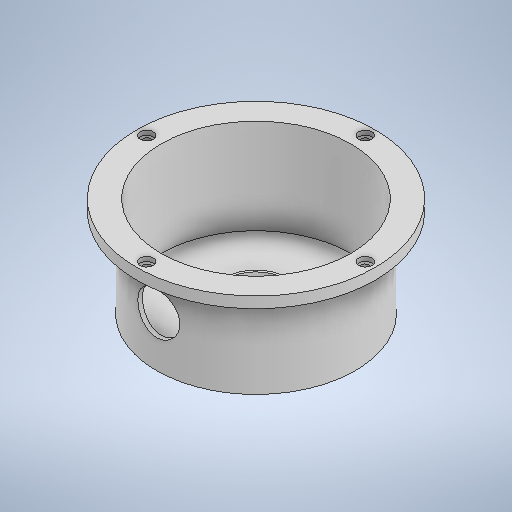
# Autodesk Inventor part: Pieza 3
Saved by Autodesk Inventor 2025.1 (Build 291241000, 241)
## iProperties
Created: 2024-08-11
Part Number: Pieza 3
Material: Genérico
Document SubType Name: Modeling
Designer: andre
Density: 1 g/cm^3
Appearance: Valor por defecto
Author: andre
Autodesk Inventor part; units mm, degrees
ref_plane "YZ Plane" through (0, 0, 0) normal (1, 0, 0) x (0, 1, 0)
ref_plane "XZ Plane" through (0, 0, 0) normal (0, 1, 0) x (-1, 0, 0)
ref_plane "XY Plane" through (0, 0, 0) normal (0, 0, 1) x (1, 0, 0)
sketch "Boceto1" plane through (0, 0, 0) normal (0, 1, 0) x (-1, 0, 0)
  circle A0 centre (0, 0) radius 45
  circle A1 centre (0, 0) radius 54
  circle A2 centre (0, 0) radius 43
  dimension "d0" = 90
  dimension "d1" = 9
  dimension "d8" = 2
  constraints: 3 centre point, 1 coincident
  measures "d0" diameter of A0
  measures "d1" radial gap between concentric circles of A0 A1
  measures "d8" radial gap between concentric circles of A0 A2
extrude "Extrusión1" add sketch "Boceto1" along normal blind 5 contours A0 | A1
sketch "Boceto2" plane through (0, 0, 0) normal (0, -1, 0) x (1, 0, 0)
  circle A0 centre (0, 0) radius 45
  circle A1 centre (0, 0) radius 43
  dimension "d7" = 2
  constraints: 2 centre point
  measures "d7" radial gap between concentric circles of A0 A1
extrude "Extrusión2" add sketch "Boceto2" along normal blind 38
sketch "Boceto3" plane through (0, -38, 0) normal (0, -1, 0) x (1, 0, 0)
  circle A0 centre (0, 0) radius 45
  constraints: 1 centre point, 1 coincident
extrude "Extrusión3" add sketch "Boceto3" along normal blind 2
sketch "Boceto4" plane through (0, 5, 0) normal (0, 1, 0) x (1, 0, 0)
  circle A0 centre (0, 0) radius 45 construction
  circle A1 centre (0, 0) radius 49.5 construction
  circle A2 centre (-49.5, 0) radius 1.625
  circle A3 centre (0, 49.5) radius 1.625
  circle A4 centre (49.5, 0) radius 1.625
  circle A5 centre (0, -49.5) radius 1.625
  dimension "d11" = 4.5
  dimension "d12" = 90
  dimension "d13" = 3.25
  dimension "d14" = 3.25
  dimension "d15" = 3.25
  dimension "d16" = 3.25
  constraints: 6 centre point, 4 point on circle, 1 coincident
  measures "d11" radial gap between concentric circles of A0 A1
  measures "d12" diameter of A0
  measures "d13" diameter of A2
  measures "d14" diameter of A3
  measures "d15" diameter of A4
  measures "d16" diameter of A5
extrude "Extrusión4" cut sketch "Boceto4" against normal blind 10
sketch "Boceto5" plane through (0, 5, 0) normal (0, 1, 0) x (1, 0, 0)
  circle A0 centre (0, 49.5) radius 1.625 projected
  circle A1 centre (0, 49.5) radius 3
  circle A2 centre (49.5, 0) radius 1.625 projected
  circle A3 centre (49.5, 0) radius 3
  circle A4 centre (0, -49.5) radius 1.625 projected
  circle A5 centre (0, -49.5) radius 3
  circle A6 centre (-49.5, 0) radius 1.625 projected
  circle A7 centre (-49.5, 0) radius 3
  point P0 (0, 0)
  dimension "d19" = 6
  dimension "d20" = 6
  dimension "d21" = 6
  dimension "d22" = 6
  constraints: 4 centre point, 4 coincident
  measures "d19" diameter of A1
  measures "d20" diameter of A3
  measures "d21" diameter of A5
  measures "d22" diameter of A7
extrude "Extrusión5" cut sketch "Boceto5" against normal blind 2 contours A0 | A1 | A2 | A3 | A4 | A5 | A6 | A7
sketch "Boceto6" plane through (0, -40, 0) normal (0, -1, 0) x (1, 0, 0)
  circle A0 centre (0, 0) radius 13.125
  dimension "d33" = 26.25
  constraints: 1 centre point, 1 coincident
  measures "d33" diameter of A0
extrude "Extrusión6" cut sketch "Boceto6" against normal blind 5
sketch "Boceto7" plane through (0, -38, 0) normal (0, 1, 0) x (1, 0, 0)
  circle A0 centre (0, 0) radius 13.125
  circle A1 centre (0, 0) radius 14.125
  dimension "d36" = 1
  dimension "d37" = 26.25
  constraints: 2 centre point, 1 coincident
  measures "d36" radial gap between concentric circles of A0 A1
  measures "d37" diameter of A0
extrude "Extrusión7" add sketch "Boceto7" along normal blind 5
fillet "Empalme de cara1" radius 5 1 edges at (-14.125, -38, 0)
sketch "Boceto8" plane through (0, -40, 0) normal (0, -1, 0) x (1, 0, 0)
  line L0 (-102.7174, -0.1449) -> (97.2826, -0.1449)
  line L1 (97.2826, -0.1449) -> (97.2826, -10.1449)
  line L2 (97.2826, -10.1449) -> (-102.7174, -10.1449)
  line L3 (-102.7174, -10.1449) -> (-102.7174, -0.1449)
  point P0 (0, 0)
  dimension "d43" = 200
  dimension "d44" = 10
  constraints: 8 end point, 2 parallel, 1 horizontal, 1 perpendicular
  measures "d43" distance of L1.end L2.end
  measures "d44" distance of L0.end L1.end
extrude "Extrusión8" add sketch "Boceto8" along normal blind 10
sketch "Boceto10" plane through (-102.7174, -40, -0.1449) normal (0, 0, 1) x (1, 0, 0)
  line L0 (57.7176, 0) -> (0, 0) projected
  line L1 (0, 0) -> (212.0347, 0)
  line L2 (156.7174, 45) -> (48.7174, 45) projected
  line L3 (48.7174, 45) -> (156.7174, 45)
  line L4 (102.7174, 45) -> (102.7174, 0) construction
  circle A0 centre (102.7174, 22.5) radius 9.55
  point P0 (102.7174, 40)
  dimension "d45" = 19.1
  constraints: 6 end point, 2 midpoint, 1 centre point, 1 coincident, 1 collinear, 1 horizontal, 1 perpendicular, 1 point on line
  measures "d45" diameter of A0
extrude "Extrusión9" cut sketch "Boceto10" along normal blind 70
sketch "Boceto11" plane through (0, -50, 0) normal (0, -1, 0) x (1, 0, 0)
  line L0 (-102.7174, -0.1449) -> (-102.7174, -10.1449) projected
  line L1 (-102.7174, -10.1449) -> (97.2826, -10.1449) projected
  line L2 (-102.7174, -0.1449) -> (97.2826, -0.1449)
  line L3 (97.2826, -0.1449) -> (97.2826, -10.1449)
  line L4 (97.2826, -10.1449) -> (-102.7174, -10.1449)
  line L5 (-102.7174, -10.1449) -> (-102.7174, -0.1449)
  point P0 (0, 0)
  constraints: 8 end point, 2 parallel, 1 horizontal, 1 perpendicular
extrude "Extrusión10" cut sketch "Boceto11" against normal blind 10
